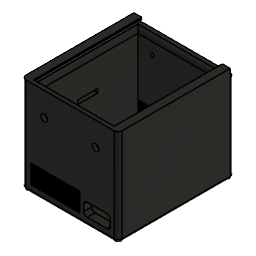
Bottom-Case (Autodesk Fusion 360 design; units mm, degrees)
part number: 2026-05-07-22-54-54-355
Autodesk Fusion 360 part; units mm, degrees
sketch "Sketch21" plane through (0, 0, 0) normal (0, 0, 1) x (1, 0, 0)
  line L0 (3, 0) -> (70, 0)
  line L1 (73, 3) -> (73, 85)
  line L2 (70, 88) -> (3, 88)
  line L3 (0, 85) -> (0, 3)
  arc A0 (0, 3) -> (3, 0) centre (3, 3) ccw
  arc A1 (70, 0) -> (73, 3) centre (70, 3) ccw
  arc A2 (73, 85) -> (70, 88) centre (70, 85) ccw
  arc A3 (3, 88) -> (0, 85) centre (3, 85) ccw
  point P0 (73, 0)
  point P1 (0, 88)
  dimension "d128" = 73
  dimension "d129" = 88
  dimension "d130" = 3
  constraint horizontal L0
  constraint vertical L1
  constraint horizontal L2
  constraint vertical L3
  constraint coincident origin L0
  constraint coincident origin L3
  constraint tangent L0 A0
  constraint tangent L3 A0
  constraint coincident P0 L0
  constraint coincident P0 L1
  constraint tangent L0 A1
  constraint tangent L1 A1
  constraint equal A0 A1
  constraint tangent L1 A2
  constraint tangent L2 A2
  constraint equal A0 A2
  constraint coincident P1 L2
  constraint coincident P1 L3
  constraint tangent L2 A3
  constraint tangent L3 A3
  constraint equal A0 A3
  measures "d128" distance of origin P0
  measures "d129" distance of origin P1
  measures "d130" radius of A0
extrude "Extrude20" add sketch "Sketch21" along normal blind 6
sketch "Sketch22" plane through (0, 0, 6) normal (0, 0, 1) x (-1, 0, 0)
  arc A0 (-3, -88) -> (0, -85) centre (-3, -85) ccw
  line L0 (0, -85) -> (0, -3)
  arc A1 (0, -3) -> (-3, 0) centre (-3, -3) ccw
  line L1 (-3, 0) -> (-70, 0)
  arc A2 (-70, 0) -> (-73, -3) centre (-70, -3) ccw
  line L2 (-73, -3) -> (-73, -85)
  arc A3 (-73, -85) -> (-70, -88) centre (-70, -85) ccw
  line L3 (-70, -88) -> (-3, -88)
  line L4 (-6, -82) -> (-67, -82)
  line L5 (-67, -82) -> (-67, -6)
  line L6 (-67, -6) -> (-6, -6)
  line L7 (-6, -6) -> (-6, -82)
  dimension "d133" = 61
  dimension "d134" = 76
  dimension "d135" = 6
  dimension "d136" = 6
  constraint horizontal L4
  constraint vertical L5
  constraint horizontal L6
  constraint vertical L7
  measures "d133" distance of L4.start L4.end
  measures "d134" distance of L4.start L6.end
  measures "d135" distance of L0 L7
  measures "d136" distance of L3 L4
extrude "Extrude21" add sketch "Sketch22" along normal blind 67.8
fillet "Fillet4" radius 3 8 edges at (36.5, 0, 0) (72.1213, 0.8787, 0) (73, 44, 0) (72.1213, 87.1213, 0) (36.5, 88, 0) (0.8787, 87.1213, 0) (0, 44, 0) (0.8787, 0.8787, 0)
sketch "Sketch23" plane through (0, 88, 0) normal (0, 1, 0) x (-1, 0, 0)
  line L0 (-70, 3) -> (-3, 3)
  line L1 (-3, 3) -> (-3, 73.8)
  line L2 (-3, 73.8) -> (-70, 73.8)
  line L3 (-70, 73.8) -> (-70, 3)
  line L4 (-67, 73.8) -> (-6, 73.8)
  line L5 (-6, 73.8) -> (-6, 67.8)
  line L6 (-6, 67.8) -> (-67, 67.8)
  line L7 (-67, 67.8) -> (-67, 73.8)
  line L8 (-73, 3) -> (-73, 73.8)
  line L9 (-67, 67.8) -> (-70, 67.8)
  line L10 (-70, 67.8) -> (-70, 70.8)
  line L11 (-70, 70.8) -> (-67, 70.8)
  line L12 (-67, 70.8) -> (-67, 67.8)
  line L13 (-6, 67.8) -> (-3, 67.8)
  line L14 (-3, 67.8) -> (-3, 70.8)
  line L15 (-3, 70.8) -> (-6, 70.8)
  line L16 (-6, 70.8) -> (-6, 67.8)
  dimension "d141" = 61
  dimension "d142" = 6
  dimension "d143" = 6
  dimension "d144" = 3
  constraint horizontal L4
  constraint vertical L5
  constraint horizontal L6
  constraint vertical L7
  constraint coincident L2 L4.start
  constraint horizontal L9
  constraint vertical L10
  constraint horizontal L11
  constraint vertical L12
  constraint horizontal L13
  constraint vertical L14
  constraint horizontal L15
  constraint vertical L16
  constraint coincident L1 L14.end
  measures "d141" distance of L4.start L4.end
  measures "d142" distance of L4.start L6.end
  measures "d143" distance of L7 L8
  measures "d144" distance of L6.end L11.end
extrude "Extrude22" cut sketch "Sketch23" against normal blind 85 contours L3 L7 L9 L10 L11 L12 | L1 L5 L13 L14 L15 L16 | L2 L4 L5 L6 L7 L12 L16
sketch "Sketch24" plane through (0, 0, 0) normal (-1, 0, 0) x (0, -1, 0)
  line L0 (-85, 3) -> (-3, 3)
  line L1 (-3, 3) -> (-3, 73.8)
  line L2 (-3, 73.8) -> (-85, 73.8)
  line L3 (-85, 73.8) -> (-85, 3)
  line L4 (-51.504, 43.8) -> (-36.504, 43.8)
  line L5 (-36.504, 43.8) -> (-36.504, 40.8)
  line L6 (-36.504, 40.8) -> (-51.504, 40.8)
  line L7 (-51.504, 40.8) -> (-51.504, 43.8)
  dimension "d147" = 15
  dimension "d148" = 3
  dimension "d150" = 33.496
  dimension "d213" = 37.8
  constraint horizontal L4
  constraint vertical L5
  constraint horizontal L6
  constraint vertical L7
  measures "d147" distance of L4.start L4.end
  measures "d148" distance of L4.start L6.end
  measures "d150" distance of L3 L7
  measures "d213" distance of L0 L6
extrude "Extrude23" cut sketch "Sketch24" against normal blind 40 contours L4 L5 L6 L7
sketch "Sketch25" plane through (0, 0, 0) normal (-1, 0, 0) x (0, -1, 0)
  line L0 (-36.504, 43.8) -> (-36.504, 40.8)
  line L1 (-36.504, 40.8) -> (-51.504, 40.8)
  line L2 (-51.504, 40.8) -> (-51.504, 43.8)
  line L3 (-51.504, 43.8) -> (-36.504, 43.8)
  line L4 (-85, 3) -> (-3, 3)
  line L5 (-3, 3) -> (-3, 73.8)
  line L6 (-3, 73.8) -> (-85, 73.8)
  line L7 (-85, 73.8) -> (-85, 3)
fillet "Fillet5" offset 6 second offset 2.5 1 edges at (0, 44.004, 40.8) measured on face at (0, 41.5013, 15.6)
fillet "Fillet6" offset 3 second offset 3 1 edges at (0, 44.004, 43.8) measured on face at (0, 14.168, 37.2)
sketch "Sketch26" plane through (0, 0, 0) normal (0, -1, 0) x (1, 0, 0)
  line L0 (3, 3) -> (70, 3)
  line L1 (70, 3) -> (70, 73.8)
  line L2 (70, 73.8) -> (3, 73.8)
  line L3 (3, 73.8) -> (3, 3)
  line L4 (64.5, 16.8) -> (49.5, 16.8)
  line L5 (47, 14.3) -> (47, 9.3)
  line L6 (49.5, 6.8) -> (64.5, 6.8)
  line L7 (67, 9.3) -> (67, 14.3)
  arc A0 (49.5, 16.8) -> (47, 14.3) centre (49.5, 14.3) ccw
  arc A1 (47, 9.3) -> (49.5, 6.8) centre (49.5, 9.3) ccw
  arc A2 (64.5, 6.8) -> (67, 9.3) centre (64.5, 9.3) ccw
  arc A3 (67, 14.3) -> (64.5, 16.8) centre (64.5, 14.3) ccw
  point P0 (67, 16.8)
  point P1 (47, 16.8)
  point P2 (67, 6.8)
  dimension "d159" = 20
  dimension "d160" = 10
  dimension "d161" = 3.8
  dimension "d198" = 2.5
  constraint horizontal L4
  constraint vertical L5
  constraint horizontal L6
  constraint vertical L7
  constraint coincident P1 L4
  constraint coincident P1 L5
  constraint tangent L4 A0
  constraint tangent L5 A0
  constraint tangent L5 A1
  constraint tangent L6 A1
  constraint equal A0 A1
  constraint coincident P2 L6
  constraint coincident P2 L7
  constraint tangent L6 A2
  constraint tangent L7 A2
  constraint equal A0 A2
  constraint coincident P0 L4
  constraint coincident P0 L7
  constraint tangent L4 A3
  constraint tangent L7 A3
  constraint equal A0 A3
  measures "d159" distance of P0 P1
  measures "d160" distance of P0 P2
  measures "d161" distance of L0 L6
  measures "d198" radius of A0
extrude "Extrude24" cut sketch "Sketch26" against normal blind 10 contours L4 L5 L6 L7 A0 A1 A2 A3
sketch "Sketch27" plane through (0, 0, 0) normal (0, -1, 0) x (1, 0, 0)
  line L0 (49.5, 16.8) -> (64.5, 16.8)
  line L1 (67, 14.3) -> (67, 9.3)
  line L2 (64.5, 6.8) -> (49.5, 6.8)
  line L3 (47, 9.3) -> (47, 14.3)
  line L4 (3, 3) -> (70, 3)
  line L5 (70, 3) -> (70, 73.8)
  line L6 (70, 73.8) -> (3, 73.8)
  line L7 (3, 73.8) -> (3, 3)
  circle A0 centre (17, 55.8) radius 1.4
  circle A1 centre (17, 55.8) radius 2.5
  circle A2 centre (56, 55.8) radius 1.4
  circle A3 centre (56, 55.8) radius 2.5
  arc A4 (67, 14.3) -> (64.5, 16.8) centre (64.5, 14.3) ccw
  arc A5 (64.5, 6.8) -> (67, 9.3) centre (64.5, 9.3) ccw
  arc A6 (47, 9.3) -> (49.5, 6.8) centre (49.5, 9.3) ccw
  arc A7 (49.5, 16.8) -> (47, 14.3) centre (49.5, 14.3) ccw
  dimension "d164" = 2.8
  dimension "d165" = 5
  dimension "d167" = 14
  dimension "d168" = 2.8
  dimension "d169" = 5
  dimension "d170" = 14
  dimension "d209" = 52.8
  dimension "d210" = 52.8
  constraint concentric A0 A1
  constraint concentric A2 A3
  measures "d164" diameter of A0
  measures "d165" diameter of A1
  measures "d167" distance of L7 A0.centre
  measures "d168" diameter of A2
  measures "d169" diameter of A3
  measures "d170" distance of L5 A2.centre
  measures "d209" distance of L4 A0.centre
  measures "d210" distance of L4 A2.centre
extrude "Extrude25" cut sketch "Sketch27" against normal blind 6 contours A0 | A2
extrude "Extrude26" cut sketch "Sketch27" against normal blind 3 contours A1 | A3
sketch "Sketch28" plane through (0, 88, 0) normal (0, 1, 0) x (-1, 0, 0)
  line L0 (-3, 67.8) -> (-70, 67.8)
  line L1 (-70, 67.8) -> (-70, 3)
  line L2 (-70, 3) -> (-3, 3)
  line L3 (-3, 3) -> (-3, 67.8)
  circle A0 centre (-56, 55.8) radius 1.4
  circle A1 centre (-56, 55.8) radius 2.5
  circle A2 centre (-17, 55.8) radius 1.4
  circle A3 centre (-17, 55.8) radius 2.5
  dimension "d176" = 2.8
  dimension "d177" = 5
  dimension "d179" = 14
  dimension "d180" = 2.8
  dimension "d181" = 5
  dimension "d182" = 14
  dimension "d211" = 52.8
  dimension "d212" = 52.8
  constraint concentric A0 A1
  constraint concentric A2 A3
  measures "d176" diameter of A0
  measures "d177" diameter of A1
  measures "d179" distance of L1 A0.centre
  measures "d180" diameter of A2
  measures "d181" diameter of A3
  measures "d182" distance of L3 A2.centre
  measures "d211" distance of L2 A0.centre
  measures "d212" distance of L2 A2.centre
extrude "Extrude30" cut sketch "Sketch28" against normal blind 6 contours A2
extrude "Extrude31" cut sketch "Sketch28" against normal blind 3 contours A1 | A3
extrude "Extrude32" cut sketch "Sketch28" against normal blind 6 contours A0
sketch "Sketch29" plane through (0, 0, 73.8) normal (0, 0, 1) x (-1, 0, 0)
  line L0 (-6, -3) -> (-6, -88)
  line L1 (-6, -88) -> (-3, -88)
  arc A0 (-3, -88) -> (0, -85) centre (-3, -85) ccw
  line L2 (0, -85) -> (0, -3)
  arc A1 (0, -3) -> (-3, 0) centre (-3, -3) ccw
  line L3 (-3, 0) -> (-70, 0)
  arc A2 (-70, 0) -> (-73, -3) centre (-70, -3) ccw
  line L4 (-73, -3) -> (-73, -85)
  arc A3 (-73, -85) -> (-70, -88) centre (-70, -85) ccw
  line L5 (-70, -88) -> (-67, -88)
  line L6 (-67, -88) -> (-67, -3)
  line L7 (-67, -3) -> (-6, -3)
  line L8 (-73, -85) -> (0, -85)
  line L9 (0, -85) -> (0, -88)
  line L10 (0, -88) -> (-73, -88)
  line L11 (-73, -88) -> (-73, -85)
  constraint horizontal L8
  constraint vertical L9
  constraint horizontal L10
  constraint vertical L11
  constraint coincident L4.end A3.start
extrude "Extrude33" cut sketch "Sketch29" against normal blind 6 contours L0 L1 A0 L8 L10 | L0 L6 L8 L10 | A3 L5 L6 L8 L10
sketch "Sketch30" plane through (0, 0, 0) normal (0, -1, 0) x (1, 0, 0)
  circle A0 centre (17, 55.8) radius 2.5
  circle A1 centre (56, 55.8) radius 2.5
  line L0 (49.5, 16.8) -> (64.5, 16.8)
  arc A2 (67, 14.3) -> (64.5, 16.8) centre (64.5, 14.3) ccw
  line L1 (67, 14.3) -> (67, 9.3)
  arc A3 (64.5, 6.8) -> (67, 9.3) centre (64.5, 9.3) ccw
  line L2 (64.5, 6.8) -> (49.5, 6.8)
  arc A4 (47, 9.3) -> (49.5, 6.8) centre (49.5, 9.3) ccw
  line L3 (47, 9.3) -> (47, 14.3)
  arc A5 (49.5, 16.8) -> (47, 14.3) centre (49.5, 14.3) ccw
  line L4 (3, 3) -> (70, 3)
  line L5 (70, 3) -> (70, 73.8)
  line L6 (70, 73.8) -> (3, 73.8)
  line L7 (3, 73.8) -> (3, 3)
  line L8 (44, 6.5) -> (7.5, 6.5)
  line L9 (7, 7) -> (7, 21.5)
  line L10 (7, 21.5) -> (44, 21.5)
  line L11 (44, 21.5) -> (44, 6.5)
  line L12 (7, 21.5) -> (7.5, 21.5)
  line L13 (8, 21) -> (8, 7)
  line L14 (7.5, 6.5) -> (7, 6.5)
  line L15 (7, 6.5) -> (7, 21.5)
  line L16 (10, 7) -> (10, 21)
  line L17 (9, 21) -> (9, 7)
  line L18 (12, 21) -> (12, 7)
  line L19 (11, 7) -> (11, 21)
  line L20 (14, 21) -> (14, 7)
  line L21 (13, 7) -> (13, 21)
  line L22 (16, 7) -> (16, 21)
  line L23 (15, 21) -> (15, 7)
  line L24 (18, 21) -> (18, 7)
  line L25 (17, 7) -> (17, 21)
  line L26 (20, 7) -> (20, 21)
  line L27 (19, 21) -> (19, 7)
  line L28 (22, 21) -> (22, 7)
  line L29 (21, 7) -> (21, 21)
  line L30 (24, 7) -> (24, 21)
  line L31 (23, 21) -> (23, 7)
  line L32 (26, 21) -> (26, 7)
  line L33 (25, 7) -> (25, 21)
  line L34 (28, 7) -> (28, 21)
  line L35 (27, 21) -> (27, 7)
  line L36 (30, 21) -> (30, 7)
  line L37 (29, 7) -> (29, 21)
  line L38 (32, 7) -> (32, 21)
  line L39 (31, 21) -> (31, 7)
  line L40 (34, 21) -> (34, 7)
  line L41 (33, 7) -> (33, 21)
  line L42 (36, 7) -> (36, 21)
  line L43 (35, 21) -> (35, 7)
  line L44 (38, 21) -> (38, 7)
  line L45 (37, 7) -> (37, 21)
  line L46 (40, 7) -> (40, 21)
  line L47 (39, 21) -> (39, 7)
  line L48 (42, 21) -> (42, 7)
  line L49 (41, 7) -> (41, 21)
  line L50 (44, 7) -> (44, 21.5)
  line L51 (44, 21.5) -> (43.5, 21.5)
  line L52 (43, 21) -> (43, 7)
  arc A6 (9.5, 21.5) -> (9, 21) centre (9.5, 21) ccw
  arc A7 (10, 21) -> (9.5, 21.5) centre (9.5, 21) ccw
  arc A8 (9, 7) -> (9.5, 6.5) centre (9.5, 7) ccw
  arc A9 (9.5, 6.5) -> (10, 7) centre (9.5, 7) ccw
  arc A10 (11, 7) -> (11.5, 6.5) centre (11.5, 7) ccw
  arc A11 (11.5, 6.5) -> (12, 7) centre (11.5, 7) ccw
  arc A12 (13, 7) -> (13.5, 6.5) centre (13.5, 7) ccw
  arc A13 (13.5, 6.5) -> (14, 7) centre (13.5, 7) ccw
  arc A14 (15, 7) -> (15.5, 6.5) centre (15.5, 7) ccw
  arc A15 (15.5, 6.5) -> (16, 7) centre (15.5, 7) ccw
  arc A16 (17, 7) -> (17.5, 6.5) centre (17.5, 7) ccw
  arc A17 (17.5, 6.5) -> (18, 7) centre (17.5, 7) ccw
  arc A18 (19, 7) -> (19.5, 6.5) centre (19.5, 7) ccw
  arc A19 (19.5, 6.5) -> (20, 7) centre (19.5, 7) ccw
  arc A20 (11.5, 21.5) -> (11, 21) centre (11.5, 21) ccw
  arc A21 (12, 21) -> (11.5, 21.5) centre (11.5, 21) ccw
  arc A22 (13.5, 21.5) -> (13, 21) centre (13.5, 21) ccw
  arc A23 (14, 21) -> (13.5, 21.5) centre (13.5, 21) ccw
  arc A24 (15.5, 21.5) -> (15, 21) centre (15.5, 21) ccw
  arc A25 (16, 21) -> (15.5, 21.5) centre (15.5, 21) ccw
  arc A26 (17.5, 21.5) -> (17, 21) centre (17.5, 21) ccw
  arc A27 (18, 21) -> (17.5, 21.5) centre (17.5, 21) ccw
  arc A28 (19.5, 21.5) -> (19, 21) centre (19.5, 21) ccw
  arc A29 (20, 21) -> (19.5, 21.5) centre (19.5, 21) ccw
  arc A30 (21.5, 21.5) -> (21, 21) centre (21.5, 21) ccw
  arc A31 (22, 21) -> (21.5, 21.5) centre (21.5, 21) ccw
  arc A32 (23.5, 21.5) -> (23, 21) centre (23.5, 21) ccw
  arc A33 (24, 21) -> (23.5, 21.5) centre (23.5, 21) ccw
  arc A34 (25.5, 21.5) -> (25, 21) centre (25.5, 21) ccw
  arc A35 (26, 21) -> (25.5, 21.5) centre (25.5, 21) ccw
  arc A36 (27.5, 21.5) -> (27, 21) centre (27.5, 21) ccw
  arc A37 (28, 21) -> (27.5, 21.5) centre (27.5, 21) ccw
  arc A38 (29.5, 21.5) -> (29, 21) centre (29.5, 21) ccw
  arc A39 (30, 21) -> (29.5, 21.5) centre (29.5, 21) ccw
  arc A40 (31.5, 21.5) -> (31, 21) centre (31.5, 21) ccw
  arc A41 (32, 21) -> (31.5, 21.5) centre (31.5, 21) ccw
  arc A42 (33.5, 21.5) -> (33, 21) centre (33.5, 21) ccw
  arc A43 (34, 21) -> (33.5, 21.5) centre (33.5, 21) ccw
  arc A44 (35.5, 21.5) -> (35, 21) centre (35.5, 21) ccw
  arc A45 (36, 21) -> (35.5, 21.5) centre (35.5, 21) ccw
  arc A46 (21, 7) -> (21.5, 6.5) centre (21.5, 7) ccw
  arc A47 (21.5, 6.5) -> (22, 7) centre (21.5, 7) ccw
  arc A48 (23, 7) -> (23.5, 6.5) centre (23.5, 7) ccw
  arc A49 (23.5, 6.5) -> (24, 7) centre (23.5, 7) ccw
  arc A50 (25, 7) -> (25.5, 6.5) centre (25.5, 7) ccw
  arc A51 (25.5, 6.5) -> (26, 7) centre (25.5, 7) ccw
  arc A52 (27, 7) -> (27.5, 6.5) centre (27.5, 7) ccw
  arc A53 (27.5, 6.5) -> (28, 7) centre (27.5, 7) ccw
  arc A54 (29, 7) -> (29.5, 6.5) centre (29.5, 7) ccw
  arc A55 (29.5, 6.5) -> (30, 7) centre (29.5, 7) ccw
  arc A56 (31, 7) -> (31.5, 6.5) centre (31.5, 7) ccw
  arc A57 (31.5, 6.5) -> (32, 7) centre (31.5, 7) ccw
  arc A58 (33, 7) -> (33.5, 6.5) centre (33.5, 7) ccw
  arc A59 (33.5, 6.5) -> (34, 7) centre (33.5, 7) ccw
  arc A60 (35, 7) -> (35.5, 6.5) centre (35.5, 7) ccw
  arc A61 (35.5, 6.5) -> (36, 7) centre (35.5, 7) ccw
  arc A62 (37, 7) -> (37.5, 6.5) centre (37.5, 7) ccw
  arc A63 (37.5, 6.5) -> (38, 7) centre (37.5, 7) ccw
  arc A64 (39, 7) -> (39.5, 6.5) centre (39.5, 7) ccw
  arc A65 (39.5, 6.5) -> (40, 7) centre (39.5, 7) ccw
  arc A66 (37.5, 21.5) -> (37, 21) centre (37.5, 21) ccw
  arc A67 (38, 21) -> (37.5, 21.5) centre (37.5, 21) ccw
  arc A68 (39.5, 21.5) -> (39, 21) centre (39.5, 21) ccw
  arc A69 (40, 21) -> (39.5, 21.5) centre (39.5, 21) ccw
  arc A70 (41.5, 21.5) -> (41, 21) centre (41.5, 21) ccw
  arc A71 (42, 21) -> (41.5, 21.5) centre (41.5, 21) ccw
  arc A72 (41, 7) -> (41.5, 6.5) centre (41.5, 7) ccw
  arc A73 (41.5, 6.5) -> (42, 7) centre (41.5, 7) ccw
  arc A74 (43, 7) -> (43.5, 6.5) centre (43.5, 7) ccw
  arc A75 (43.5, 6.5) -> (44, 7) centre (43.5, 7) ccw
  arc A76 (43.5, 21.5) -> (43, 21) centre (43.5, 21) ccw
  arc A77 (7.5, 6.5) -> (8, 7) centre (7.5, 7) ccw
  arc A78 (8, 21) -> (7.5, 21.5) centre (7.5, 21) ccw
  arc A79 (7, 7) -> (7.5, 6.5) centre (7.5, 7) ccw
  arc A80 (7.5, 21.5) -> (7, 21) centre (7.5, 21) ccw
  arc A81 (44, 21) -> (43.5, 21.5) centre (43.5, 21) ccw
  dimension "d199" = 0.5
  constraint horizontal L8
  constraint vertical L9
  constraint horizontal L10
  constraint vertical L11
  constraint horizontal L12
  constraint vertical L13
  constraint horizontal L14
  constraint vertical L15
  constraint vertical L16
  constraint vertical L17
  constraint vertical L18
  constraint vertical L19
  constraint vertical L20
  constraint vertical L21
  constraint vertical L22
  constraint vertical L23
  constraint vertical L24
  constraint vertical L25
  constraint vertical L26
  constraint vertical L27
  constraint vertical L28
  constraint vertical L29
  constraint vertical L30
  constraint vertical L31
  constraint vertical L32
  constraint vertical L33
  constraint vertical L34
  constraint vertical L35
  constraint vertical L36
  constraint vertical L37
  constraint vertical L38
  constraint vertical L39
  constraint vertical L40
  constraint vertical L41
  constraint vertical L42
  constraint vertical L43
  constraint vertical L44
  constraint vertical L45
  constraint vertical L46
  constraint vertical L47
  constraint vertical L48
  constraint vertical L49
  constraint vertical L50
  constraint horizontal L51
  constraint vertical L52
  constraint tangent L17 A6
  constraint tangent L16 A7
  constraint equal A6 A7
  constraint coincident A6.start A7.end
  constraint tangent L17 A8
  constraint equal A6 A8
  constraint tangent L16 A9
  constraint equal A6 A9
  constraint coincident A8.end A9.start
  constraint tangent L19 A10
  constraint equal A6 A10
  constraint tangent L18 A11
  constraint equal A6 A11
  constraint coincident A10.end A11.start
  constraint tangent L21 A12
  constraint equal A6 A12
  constraint tangent L20 A13
  constraint equal A6 A13
  constraint coincident A12.end A13.start
  constraint tangent L23 A14
  constraint equal A6 A14
  constraint tangent L22 A15
  constraint equal A6 A15
  constraint coincident A14.end A15.start
  constraint tangent L25 A16
  constraint equal A6 A16
  constraint tangent L24 A17
  constraint equal A6 A17
  constraint coincident A16.end A17.start
  constraint tangent L27 A18
  constraint equal A6 A18
  constraint tangent L26 A19
  constraint equal A6 A19
  constraint coincident A18.end A19.start
  constraint tangent L19 A20
  constraint equal A6 A20
  constraint tangent L18 A21
  constraint equal A6 A21
  constraint coincident A20.start A21.end
  constraint tangent L21 A22
  constraint equal A6 A22
  constraint tangent L20 A23
  constraint equal A6 A23
  constraint coincident A22.start A23.end
  constraint tangent L23 A24
  constraint equal A6 A24
  constraint tangent L22 A25
  constraint equal A6 A25
  constraint coincident A24.start A25.end
  constraint tangent L25 A26
  constraint equal A6 A26
  constraint tangent L24 A27
  constraint equal A6 A27
  constraint coincident A26.start A27.end
  constraint tangent L27 A28
  constraint equal A6 A28
  constraint tangent L26 A29
  constraint equal A6 A29
  constraint coincident A28.start A29.end
  constraint tangent L29 A30
  constraint equal A6 A30
  constraint tangent L28 A31
  constraint equal A6 A31
  constraint coincident A30.start A31.end
  constraint tangent L31 A32
  constraint equal A6 A32
  constraint tangent L30 A33
  constraint equal A6 A33
  constraint coincident A32.start A33.end
  constraint tangent L33 A34
  constraint equal A6 A34
  constraint tangent L32 A35
  constraint equal A6 A35
  constraint coincident A34.start A35.end
  constraint tangent L35 A36
  constraint equal A6 A36
  constraint tangent L34 A37
  constraint equal A6 A37
  constraint coincident A36.start A37.end
  constraint tangent L37 A38
  constraint equal A6 A38
  constraint tangent L36 A39
  constraint equal A6 A39
  constraint coincident A38.start A39.end
  constraint tangent L39 A40
  constraint equal A6 A40
  constraint tangent L38 A41
  constraint equal A6 A41
  constraint coincident A40.start A41.end
  constraint tangent L41 A42
  constraint equal A6 A42
  constraint tangent L40 A43
  constraint equal A6 A43
  constraint coincident A42.start A43.end
  constraint tangent L43 A44
  constraint equal A6 A44
  constraint tangent L42 A45
  constraint equal A6 A45
  constraint coincident A44.start A45.end
  constraint tangent L29 A46
  constraint equal A6 A46
  constraint tangent L28 A47
  constraint equal A6 A47
  constraint coincident A46.end A47.start
  constraint tangent L31 A48
  constraint equal A6 A48
  constraint tangent L30 A49
  constraint equal A6 A49
  constraint coincident A48.end A49.start
  constraint tangent L33 A50
  constraint equal A6 A50
  constraint tangent L32 A51
  constraint equal A6 A51
  constraint coincident A50.end A51.start
  constraint tangent L35 A52
  constraint equal A6 A52
  constraint tangent L34 A53
  constraint equal A6 A53
  constraint coincident A52.end A53.start
  constraint tangent L37 A54
  constraint equal A6 A54
  constraint tangent L36 A55
  constraint equal A6 A55
  constraint coincident A54.end A55.start
  constraint tangent L39 A56
  constraint equal A6 A56
  constraint tangent L38 A57
  constraint equal A6 A57
  constraint coincident A56.end A57.start
  constraint tangent L41 A58
  constraint equal A6 A58
  constraint tangent L40 A59
  constraint equal A6 A59
  constraint coincident A58.end A59.start
  constraint tangent L43 A60
  constraint equal A6 A60
  constraint tangent L42 A61
  constraint equal A6 A61
  constraint coincident A60.end A61.start
  constraint tangent L45 A62
  constraint equal A6 A62
  constraint tangent L44 A63
  constraint equal A6 A63
  constraint coincident A62.end A63.start
  constraint tangent L47 A64
  constraint equal A6 A64
  constraint tangent L46 A65
  constraint equal A6 A65
  constraint coincident A64.end A65.start
  constraint tangent L45 A66
  constraint equal A6 A66
  constraint tangent L44 A67
  constraint equal A6 A67
  constraint coincident A66.start A67.end
  constraint tangent L47 A68
  constraint equal A6 A68
  constraint tangent L46 A69
  constraint equal A6 A69
  constraint coincident A68.start A69.end
  constraint tangent L49 A70
  constraint equal A6 A70
  constraint tangent L48 A71
  constraint equal A6 A71
  constraint coincident A70.start A71.end
  constraint tangent L49 A72
  constraint equal A6 A72
  constraint tangent L48 A73
  constraint equal A6 A73
  constraint coincident A72.end A73.start
  constraint tangent L52 A74
  constraint equal A6 A74
  constraint tangent L50 A75
  constraint equal A6 A75
  constraint coincident A74.end A75.start
  constraint tangent L51 A76
  constraint tangent L52 A76
  constraint equal A6 A76
  constraint tangent L13 A77
  constraint tangent L14 A77
  constraint equal A6 A77
  constraint tangent L12 A78
  constraint tangent L13 A78
  constraint equal A6 A78
  constraint tangent L8 A79
  constraint tangent L9 A79
  constraint equal A6 A79
  constraint coincident L15 A80.end
  constraint coincident A78.centre A80.centre
  constraint coincident L11 A81.start
  constraint coincident A76.centre A81.centre
  measures "d199" radius of A6
extrude "Extrude34" cut sketch "Sketch30" against normal blind 100 contours L11 L50 L52 A74 A75 A76 A81 | L48 L49 A70 A71 A72 A73 | L46 L47 A64 A65 A68 A69 | L44 L45 A62 A63 A66 A67 | L42 L43 A44 A45 A60 A61 | L40 L41 A42 A43 A58 A59 | L38 L39 A40 A41 A56 A57 | L36 L37 A38 A39 A54 A55 | L34 L35 A36 A37 A52 A53 | L32 L33 A34 A35 A50 A51 | L30 L31 A32 A33 A48 A49 | L28 L29 A30 A31 A46 A47 | L26 L27 A18 A19 A28 A29 | L24 L25 A16 A17 A26 A27 | L22 L23 A14 A15 A24 A25 | L20 L21 A12 A13 A22 A23 | L18 L19 A10 A11 A20 A21 | L16 L17 A6 A7 A8 A9 | L9 L13 L15 A77 A78 A79 A80
sketch "Sketch31" plane through (0, 0, 6) normal (0, 0, 1) x (-1, 0, 0)
  line L0 (-67, -6) -> (-67, -82)
  line L1 (-67, -82) -> (-6, -82)
  line L2 (-6, -82) -> (-6, -6)
  line L3 (-6, -6) -> (-67, -6)
  line L4 (-6, -82) -> (-14, -82)
  line L5 (-14, -82) -> (-14, -6)
  line L6 (-14, -6) -> (-6, -6)
  line L7 (-6, -6) -> (-6, -82)
  line L8 (-14, -6) -> (-67, -6)
  line L9 (-67, -6) -> (-67, -14)
  line L10 (-67, -14) -> (-14, -14)
  line L11 (-14, -14) -> (-14, -6)
  line L12 (-67, -14) -> (-59, -14)
  line L13 (-59, -14) -> (-59, -82)
  line L14 (-59, -82) -> (-67, -82)
  line L15 (-67, -82) -> (-67, -14)
  line L16 (-59, -82) -> (-14, -82)
  line L17 (-14, -82) -> (-14, -74)
  line L18 (-14, -74) -> (-59, -74)
  line L19 (-59, -74) -> (-59, -82)
  constraint horizontal L4
  constraint vertical L5
  constraint horizontal L6
  constraint vertical L7
  constraint coincident L3 L5.end
  constraint coincident L1.end L2.start
  constraint horizontal L8
  constraint vertical L9
  constraint horizontal L10
  constraint vertical L11
  constraint coincident L0 L9.end
  constraint horizontal L12
  constraint vertical L13
  constraint horizontal L14
  constraint vertical L15
  constraint coincident L1 L13.end
  constraint horizontal L16
  constraint vertical L17
  constraint horizontal L18
  constraint vertical L19
  constraint coincident L5 L17.end
extrude "Extrude35" cut sketch "Sketch31" against normal blind 3 contours L0 L3 L5 L8 L9 L10 L11 L12 | L0 L1 L10 L12 L13 L14 L15 L19 | L1 L2 L3 L4 L5 L6 L7 L11 L17 | L1 L5 L13 L16 L17 L18 L19
fillet "Fillet7" radius 2 2 edges at (67, 44, 70.8) (6, 44, 70.8)
fillet "Fillet8" radius 3 4 edges at (36.5, 6, 67.8) (67, 44, 67.8) (36.5, 82, 67.8) (6, 44, 67.8)
